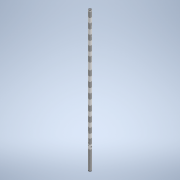
# Autodesk Inventor part: burder_rod_2
Saved by Autodesk Inventor 2020 (Build 240168000, 168)
## iProperties
Created: 2019-06-12
Part Number: burder_rod_2
Material: Generic
Document SubType Name: Modeling
Designer: ColinP
Density: 1 g/cm^3
Appearance: Default
Mass: 1.26312 g
Surface Area: 40.7053 cm^2
Volume: 1.26312 cm^3
Author: ColinP
Autodesk Inventor part; units mm, degrees
ref_plane "YZ Plane" through (0, 0, 0) normal (1, 0, 0) x (0, 1, 0)
ref_plane "XZ Plane" through (0, 0, 0) normal (0, 1, 0) x (-1, 0, 0)
ref_plane "XY Plane" through (0, 0, 0) normal (0, 0, 1) x (1, 0, 0)
sketch "Sketch1" plane through (0, 0, 0) normal (0, 1, 0) x (-1, 0, 0)
  circle A0 centre (0, 0) radius 1.5875
  dimension "d0" = 3.175
  constraints: 1 centre point, 1 coincident
  measures "d0" diameter of A0
extrude "Extrusion1" add sketch "Sketch1" along normal blind 254
sketch "Sketch9" plane through (0, 0, 0) normal (1, 0, 0) x (0, 1, 0)
  line L0 (0, -1.5875) -> (0, 1.5875) projected
  line L1 (254, -1.5875) -> (254, 1.5875) projected
  line L2 (254, 0) -> (228.6, 0)
  line L3 (0, 0) -> (25.4, 0)
  dimension "d42" = 25.4
  dimension "d43" = 25.4
  constraints: 4 end point, 2 horizontal, 1 midpoint
  measures "d42" distance of L2.start L2.end
  measures "d43" distance of L3.start L3.end
hole "Hole5" at (0, 25.4, 0) direction (-1, 0, 0) diameter 1.1906 end through all both
hole "Hole6" [suppressed]
sketch "Sketch10" plane through (0, 254, 0) normal (0, 1, 0) x (1, 0, 0)
  circle A0 centre (0, 0) radius 1.5875 projected
  constraints: 1 coincident
hole "Hole7" at (0, 254, 0) direction (0, -1, 0) diameter 1.905 end through all
thread "Thread28" size "M3.5x0.6" class "6g" standard "ISO Metric profile" length 6.35 offset 27.94
thread "Thread29" size "M3.5x0.6" class "6g" standard "ISO Metric profile" length 6.35 offset 39.878
thread "Thread30" size "M3.5x0.6" class "6g" standard "ISO Metric profile" length 6.35 offset 51.816
thread "Thread31" size "M3.5x0.6" class "6g" standard "ISO Metric profile" length 6.35 offset 63.754
thread "Thread32" size "M3.5x0.6" class "6g" standard "ISO Metric profile" length 6.35 offset 75.692
thread "Thread33" size "M3.5x0.6" class "6g" standard "ISO Metric profile" length 6.35 offset 87.63
thread "Thread34" size "M3.5x0.6" class "6g" standard "ISO Metric profile" length 6.35 offset 99.568
thread "Thread35" size "M3.5x0.6" class "6g" standard "ISO Metric profile" length 6.35 offset 111.506
thread "Thread36" size "M3.5x0.6" class "6g" standard "ISO Metric profile" length 6.35 offset 122.936
thread "Thread37" size "M3.5x0.6" class "6g" standard "ISO Metric profile" length 6.35 offset 134.112
thread "Thread38" size "M3.5x0.6" class "6g" standard "ISO Metric profile" length 22.86
thread "Thread40" size "M3.5x0.6" class "6g" standard "ISO Metric profile" length 6.35 offset 99.06
thread "Thread41" size "M3.5x0.6" class "6g" standard "ISO Metric profile" length 6.35 offset 86.995
thread "Thread42" size "5-40 UNC" class "2A" standard "ANSI Unified Screw Threads" length 6.35 offset 74.93
thread "Thread43" size "5-40 UNC" class "2A" standard "ANSI Unified Screw Threads" length 6.35 offset 62.23
thread "Thread44" size "5-40 UNC" class "2A" standard "ANSI Unified Screw Threads" length 6.35 offset 50.8
thread "Thread45" size "M3.5x0.6" class "6g" standard "ISO Metric profile" length 6.35 offset 39.37
thread "Thread46" size "M3.5x0.6" class "6g" standard "ISO Metric profile" length 6.35 offset 27.94
sketch "Sketch15" plane through (0, 254, 0) normal (0, 1, 0) x (1, 0, 0)
  circle A0 centre (0, 0) radius 1.5875 projected
  circle A1 centre (0, 0) radius 0.9525 projected
extrude "Extrusion4" cut sketch "Sketch15" against normal blind 86.36
body "Solid1"
